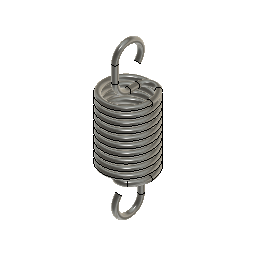
Tension Spring (Autodesk Fusion 360 design; units mm, degrees)
Autodesk Fusion 360 part; units mm, degrees
coil "CoilPrimitive1" add diameter 40 section circle size 5 on centre turns 10 pitch 6 right hand placed x (1, 0, 0) y (0, 1, 0) z (0, 0, 1) at (0, 0, 0)
ref_plane "WorkPlane1" through (0, 0, 60) normal (0, 0, 1) x (1, 0, 0)
sketch "Sketch2" plane through (0, 0, 60) normal (0, 0, 1) x (1, 0, 0)
  line L0 (0, 0) -> (0, 8.2843)
  arc A0 (14.1421, 14.1421) -> (0, 8.2843) centre (8.2843, 8.2843) ccw
  arc A1 (20, 0) -> (14.1421, 14.1421) centre (0, 0) ccw
  line L1 (22.5, 0) -> (17.5, 0)
  dimension "d8" = 45
  constraint coincident L0.start A1.centre
  constraint vertical L0
  constraint tangent L0 A0
  constraint coincident A1.start L1
  constraint midpoint A1.start L1
  constraint tangent A0 A1
  measures "d8" angle of A0.start L0.start A1.start
sweep "Sweep1" add 1 faces at (20.8421, 0, 59.0327) path "Sketch2" along A1 A0 L0
sketch "Sketch3" plane through (0, 0, 0) normal (1, 0, 0) x (0, 1, 0)
  line L0 (0, 60) -> (-38.3711, 60) construction
  arc A0 (-12, 72) -> (0, 60) centre (0, 72) ccw
  line L1 (-12, 72) -> (-12, 87)
  arc A1 (8.4853, 78.5147) -> (-12, 87) centre (0, 87) ccw
  line L2 (0, 87) -> (16.3925, 87) construction
  line L3 (0, 87) -> (10.9536, 76.0464) construction
  point P0 (0, 60)
  dimension "d15" = 45
  dimension "d16" = 12
  dimension "d17" = 15
  dimension "d18" = 12
  constraint horizontal L0
  constraint coincident P0 L0.start
  constraint tangent L0 A0
  constraint vertical L1
  constraint tangent L1 A1
  constraint tangent A0 L1
  constraint coincident A1.centre L2.start
  constraint horizontal L2
  constraint coincident A1.start L3
  measures "d15" angle of L2 L3
  measures "d16" radius of A0
  measures "d17" distance of A0.start L1.end
  measures "d18" radius of A1
sweep "Sweep2" add 1 faces at (-0.8421, 0, 59.0327) path "Sketch3" along A1 L1 A0
sketch "Sketch4" plane through (0, 0, 0) normal (0, 0, 1) x (1, 0, 0)
  line L0 (0, 0) -> (0, -8.2843)
  arc A0 (0, -8.2843) -> (14.1421, -14.1421) centre (8.2843, -8.2843) ccw
  arc A1 (14.1421, -14.1421) -> (20, 0) centre (0, 0) ccw
  line L1 (22.5, 0) -> (17.5, 0)
  dimension "d25" = 45
  constraint coincident L0.start A1.centre
  constraint vertical L0
  constraint tangent L0 A0
  constraint midpoint A1.end L1
  constraint tangent A0 A1
  measures "d25" angle of A0.end L0.start A1.end
sweep "Sweep3" add 1 faces at (20.5244, 0, -0.9455) path "Sketch4" along L0 A0 A1
sketch "Sketch6" plane through (0, 0, 0) normal (1, 0, 0) x (0, 1, 0)
  line L0 (0, 0) -> (29.213, 0) construction
  arc A0 (12, -12) -> (0, 0) centre (0, -12) ccw
  line L1 (12, -12) -> (12, -27)
  arc A1 (-8.4853, -18.5147) -> (12, -27) centre (0, -27) ccw
  line L2 (0, -27) -> (-20.3499, -27) construction
  line L3 (0, -27) -> (-15.128, -11.872) construction
  dimension "d32" = 45
  dimension "d33" = 12
  dimension "d34" = 15
  dimension "d35" = 12
  constraint coincident L0.start A0.end
  constraint horizontal L0
  constraint tangent L0 A0
  constraint vertical L1
  constraint tangent L1 A1
  constraint coincident A1.centre L2.start
  constraint perpendicular L1 L2
  constraint coincident A1.start L3
  constraint tangent A0 L1
  measures "d32" angle of L2 L3
  measures "d33" radius of A0
  measures "d34" distance of A0.start L1.end
  measures "d35" radius of A1
sweep "Sweep4" add 1 faces at (0.5651, 0, -0.5356) path "Sketch6" along A0 L1 A1
